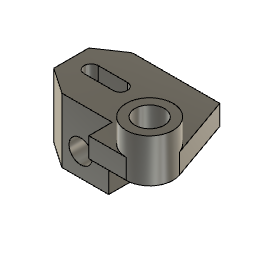
drawing_4 v1 (Autodesk Fusion 360 design; units mm, degrees)
Autodesk Fusion 360 part; units mm, degrees
note: some values were not read from the file. Set by a fixed rule: which sketch regions a step uses.
sketch "Sketch1" plane through (0, 0, 0) normal (0, 0, 1) x (1, 0, 0)
  line L0 (0, 0) -> (50, 0)
  line L1 (0, 0) -> (-25, 0)
  line L2 (-47, -30) -> (50, -30)
  line L3 (-47, -30) -> (-47, -15)
  line L4 (-47, -30) -> (-47, -45)
  line L5 (-47, -15) -> (-25, 0)
  line L6 (-25, 0) -> (-25, -30)
  line L7 (-25, -30) -> (-25, -60)
  line L8 (-25, -60) -> (-47, -45)
  line L9 (-25, -60) -> (18, -60)
  line L10 (18, -60) -> (18, -30)
  line L11 (50, -30) -> (50, -60)
  circle A0 centre (50, -60) radius 12.5
  circle A1 centre (50, -60) radius 20
  line L12 (18, -60) -> (18, -80)
  line L13 (18, -80) -> (50, -80)
  line L14 (50, 0) -> (68.8562, -53.3333)
  dimension "d3" = 50
  dimension "d4" = 25
  dimension "d8" = 15
  dimension "d9" = 15
  dimension "d11" = 30
  dimension "d12" = 25
  dimension "d13" = 40
  constraint coincident L0.start L1.start
  constraint horizontal L0
  constraint parallel L0 L1
  constraint perpendicular L2 L3
  constraint perpendicular L2 L4
  constraint coincident L2 L6.end
  constraint perpendicular L2 L6
  constraint perpendicular L2 L7
  constraint perpendicular L7 L9
  constraint coincident L2 L10.end
  constraint perpendicular L2 L10
  constraint perpendicular L2 L11
  constraint coincident L11.end A0.centre
  constraint concentric A0 A1
  constraint perpendicular L9 L12
  constraint coincident A1 L13.end
  constraint tangent A1 L13
  constraint perpendicular L12 L13
  constraint coincident A1 L14.end
  constraint tangent A1 L14
  measures "d3" distance of L0.start L0.end
  measures "d4" distance of L0.start L1.end
  measures "d8" distance of L2.start L3.end
  measures "d9" distance of L2.start L4.end
  measures "d11" distance of L2.end L11.end
  measures "d12" diameter of A0
  measures "d13" diameter of A1
extrude "Extrude1" add sketch "Sketch1" along normal blind 55 contours L0 L1 L2 L6 L11 A1 L14 | L2 L3 L5 L6 | A1 | L2 L4 L7 L8 | L2 L7 L9 L10 | L2 L10 L11 A1 L12 L13 | A0
sketch "Sketch2" plane through (0, -80, 0) normal (0, -1, 0) x (1, 0, 0)
  line L0 (18, 0) -> (50, 0)
  line L1 (50, 0) -> (50, 55)
  line L2 (50, 55) -> (18, 55)
  line L3 (18, 55) -> (18, 0)
  line L4 (15, -0.0176) -> (15, 34.9824)
  line L5 (15, 34.9824) -> (18, 34.9824)
  circle A0 centre (18, 34.9824) radius 3
  line L6 (18, 34.9824) -> (18, 37.9824)
  line L7 (70.6384, 36.4824) -> (70.6384, -2.3651)
  line L8 (70.6384, -2.3651) -> (18, 0)
  line L9 (18, 37.9824) -> (30, 37.9824)
  line L10 (30, 37.9824) -> (71, 37.9824)
  line L11 (71, 37.9824) -> (70.6384, 36.4824)
  dimension "d17" = 35
  dimension "d19" = 3
  dimension "d20" = 6
  constraint perpendicular L0 L4
  constraint perpendicular L3 L5
  constraint coincident L5.end A0.centre
  constraint coincident A0 L6.end
  constraint perpendicular L5 L6
  constraint parallel L1 L7
  constraint coincident L0.start L3.end
  constraint tangent A0 L9
  constraint perpendicular L1 L10
  measures "d17" distance of L4.start L4.end
  measures "d19" distance of L4.end L5.end
  measures "d20" diameter of A0
extrude "Extrude2" cut sketch "Sketch2" against normal blind 115 contours L0 L1 L3 A0 L9 L10 | L0 L1 L7 L8 L10 L11 | L3 L5 A0 | L3 A0 L6 | L3 L5 A0 L6
sketch "Sketch3" plane through (0, -60, 0) normal (0, -1, 0) x (1, 0, 0)
  arc A0 (18, 37.9824) -> (18, 31.9824) centre (18, 34.9824) ccw
  line L0 (18, 37.9824) -> (18, 55)
  line L1 (18, 55) -> (-25, 55)
  line L2 (-25, 55) -> (-25, 0)
  line L3 (-25, 0) -> (18, 0)
  line L4 (18, 0) -> (18, 31.9824)
  line L5 (15, 34.9824) -> (18, 34.9824)
  line L6 (18, 34.9824) -> (18, 0)
  line L7 (18, 0) -> (15, 0)
  line L8 (15, 0) -> (15, 34.9824)
  constraint horizontal L5
  constraint vertical L6
  constraint horizontal L7
  constraint vertical L8
  constraint coincident L3.end L4.start
  constraint midpoint A0 L5.start
extrude "Extrude3" cut sketch "Sketch3" against normal blind 120 contours A0 L3 L4 L6 L7 L8
sketch "Sketch4" plane through (0, 0, 55) normal (0, 0, 1) x (-1, 0, 0)
  line L0 (-50, 0) -> (25, 0)
  line L1 (25, 0) -> (47, 15)
  line L2 (47, 15) -> (47, 45)
  line L3 (47, 45) -> (25, 60)
  line L4 (25, 60) -> (-18, 60)
  line L5 (-18, 60) -> (-18, 80)
  line L6 (-18, 80) -> (-50, 80)
  arc A0 (-50, 80) -> (-68.8562, 53.3333) centre (-50, 60) ccw
  line L7 (-68.8562, 53.3333) -> (-50, 0)
  line L8 (-50, 80) -> (-50, 60)
  line L9 (-50, 60) -> (-70, 60)
  circle A1 centre (-50, 60) radius 12.5
  dimension "d25" = 25
  constraint coincident L6.end A0.start
  constraint coincident A0.centre L8.end
  constraint coincident A0 L9.end
  constraint perpendicular L8 L9
  measures "d25" diameter of A1
extrude "Extrude4" cut sketch "Sketch4" against normal blind 50 contours L8 L9 A1 | L8 L9 A1
sketch "Sketch5" plane through (0, 0, 55) normal (0, 0, 1) x (-1, 0, 0)
  circle A0 centre (-50, 60) radius 12.5
  line L0 (-50, 0) -> (25, 0)
  line L1 (25, 0) -> (47, 15)
  line L2 (47, 15) -> (47, 45)
  line L3 (47, 45) -> (25, 60)
  line L4 (25, 60) -> (-18, 60)
  line L5 (-18, 60) -> (-18, 80)
  line L6 (-18, 80) -> (-50, 80)
  arc A1 (-50, 80) -> (-68.8562, 53.3333) centre (-50, 60) ccw
  line L7 (-68.8562, 53.3333) -> (-50, 0)
  line L8 (47, 30) -> (47, 20)
  line L9 (47, 30) -> (47, 40)
  line L10 (47, 30) -> (30, 30)
  circle A2 centre (30, 30) radius 6
  line L11 (30, 30) -> (30, 24)
  line L12 (30, 30) -> (30, 36)
  line L13 (30, 30) -> (5, 30)
  circle A3 centre (5, 30) radius 6
  line L14 (30, 24) -> (5, 24)
  line L15 (30, 36) -> (5, 36)
  dimension "d28" = 10
  dimension "d29" = 10
  dimension "d30" = 17
  dimension "d31" = 12
  dimension "d32" = 25
  dimension "d33" = 12
  constraint midpoint L2 L8.start
  constraint perpendicular L2 L10
  constraint coincident L10.end A2.centre
  constraint coincident A2 L11.end
  constraint perpendicular L10 L11
  constraint coincident A2 L12.end
  constraint perpendicular L10 L12
  constraint perpendicular L12 L13
  constraint coincident L13.end A3.centre
  constraint coincident A3 L14.end
  constraint tangent A3 L14
  constraint coincident A3 L15.end
  constraint tangent A3 L15
  measures "d28" distance of L8.start L8.end
  measures "d29" distance of L8.start L9.end
  measures "d30" distance of L8.start L10.end
  measures "d31" diameter of A2
  measures "d32" distance of L10.end L13.end
  measures "d33" diameter of A3
extrude "Extrude5" cut sketch "Sketch5" against normal blind 20 contours L10 A2 L11 | L10 A2 L12 | A2 L12 L13 | A2 L11 L13 | A2 L13 A3 L15 | A2 L13 A3 L14 | A3
sketch "Sketch6" plane through (0, 0, 55) normal (0, 0, 1) x (-1, 0, 0)
  line L0 (5, 36) -> (30, 36)
  arc A0 (30, 24) -> (30, 36) centre (30, 30) ccw
  line L1 (30, 24) -> (5, 24)
  arc A1 (5, 36) -> (5, 24) centre (5, 30) ccw
  circle A2 centre (-50, 60) radius 12.5
  line L2 (-50, 0) -> (25, 0)
  line L3 (25, 0) -> (47, 15)
  line L4 (47, 15) -> (47, 45)
  line L5 (47, 45) -> (25, 60)
  line L6 (25, 60) -> (-18, 60)
  line L7 (-18, 60) -> (-18, 80)
  line L8 (-18, 80) -> (-50, 80)
  arc A3 (-50, 80) -> (-68.8562, 53.3333) centre (-50, 60) ccw
  line L9 (-68.8562, 53.3333) -> (-50, 0)
  circle A4 centre (-50, 60) radius 20
  circle A5 centre (-50, 60) radius 12.5
  dimension "d36" = 40
  dimension "d37" = 25
  constraint concentric A2 A4
  constraint concentric A4 A5
  measures "d36" diameter of A4
  measures "d37" diameter of A5
extrude "Extrude6" add sketch "Sketch6" along normal blind 20 contours A3 A4
sketch "Sketch7" plane through (0, -60, 0) normal (0, -1, 0) x (1, 0, 0)
  line L0 (15, 0) -> (15, 34.9824)
  arc A0 (18, 37.9824) -> (15, 34.9824) centre (18, 34.9824) ccw
  line L1 (18, 37.9824) -> (18, 55)
  line L2 (18, 55) -> (-25, 55)
  line L3 (-25, 55) -> (-25, 0)
  line L4 (-25, 0) -> (15, 0)
  line L5 (-47, 0) -> (-9, 0)
  line L6 (-9, 0) -> (-9, 20)
  circle A1 centre (-9, 20) radius 10
  dimension "d40" = 38
  dimension "d41" = 20
  dimension "d42" = 20
  constraint perpendicular L3 L5
  constraint perpendicular L4 L6
  constraint coincident L6.end A1.centre
  measures "d40" distance of L5.start L5.end
  measures "d41" distance of L5.end L6.end
  measures "d42" diameter of A1
extrude "Extrude7" cut sketch "Sketch7" against normal blind 130 contours A1
sketch "Sketch8" plane through (0, 0, 0) normal (0, 0, -1) x (1, 0, 0)
  line L0 (15, 0) -> (15, 60)
  line L1 (15, 60) -> (-25, 60)
  line L2 (-25, 60) -> (-47, 45)
  line L3 (-47, 45) -> (-47, 15)
  line L4 (-47, 15) -> (-25, 0)
  line L5 (-25, 0) -> (15, 0)
  line L6 (-47, 30) -> (15, 30)
  line L7 (-47, 30) -> (-32, 30)
  line L8 (15, 30) -> (0, 30)
  circle A0 centre (-32, 30) radius 10
  circle A1 centre (0, 30) radius 10
  dimension "d45" = 15
  dimension "d46" = 15
  dimension "d47" = 20
  dimension "d48" = 20
  constraint midpoint L3 L6.start
  constraint midpoint L0 L6.end
  constraint perpendicular L3 L7
  constraint perpendicular L0 L8
  constraint coincident L7.end A0.centre
  constraint coincident L8.end A1.centre
  measures "d45" distance of L6.start L7.end
  measures "d46" distance of L6.end L8.end
  measures "d47" diameter of A0
  measures "d48" diameter of A1
extrude "Extrude8" cut sketch "Sketch8" against normal blind 35 contours L6 L8 A1 | L6 L8 A1 | L6 L7 A0 | L6 L7 A0
equation "d34 = -55.00 mm + 35 mm"
equation "d38 = 75.00 mm - 55 mm"
